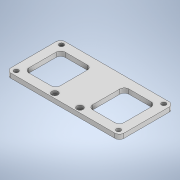
# Autodesk Inventor part: Battery_Plate
Saved by Autodesk Inventor 2021 (Build 250183000, 183)
## iProperties
Created: 2021-07-26
Part Number: Battery_Plate
Material: Generic
Document SubType Name: Modeling
Designer: rquic
Density: 1 g/cm^3
Appearance: Default
Author: rquic
Autodesk Inventor part; units mm, degrees
ref_plane "YZ Plane" through (0, 0, 0) normal (1, 0, 0) x (0, 1, 0)
ref_plane "XZ Plane" through (0, 0, 0) normal (0, 1, 0) x (-1, 0, 0)
ref_plane "XY Plane" through (0, 0, 0) normal (0, 0, 1) x (1, 0, 0)
sketch "Sketch1" plane through (0, 0, 0) normal (0, 1, 0) x (-1, 0, 0)
  line L0 (33.3375, 19.05) -> (-33.3375, 19.05)
  line L1 (-33.3375, 19.05) -> (-33.3375, -19.05)
  line L2 (-33.3375, -19.05) -> (33.3375, -19.05)
  line L3 (33.3375, -19.05) -> (33.3375, 19.05)
  line L4 (33.3375, 19.05) -> (-33.3375, -19.05) construction
  line L5 (-33.3375, 19.05) -> (33.3375, -19.05) construction
  line L6 (39.6875, -19.05) -> (-39.6875, -19.05)
  line L7 (-39.6875, -19.05) -> (-39.6875, 19.05)
  line L8 (-39.6875, 19.05) -> (39.6875, 19.05)
  line L9 (39.6875, 19.05) -> (39.6875, -19.05)
  line L10 (39.6875, -19.05) -> (-39.6875, 19.05) construction
  line L11 (-39.6875, -19.05) -> (39.6875, 19.05) construction
  circle A0 centre (35.8775, -15.875) radius 1.5875
  circle A1 centre (35.8775, 15.875) radius 1.5875
  circle A2 centre (-35.8775, -15.875) radius 1.5875
  circle A3 centre (-35.8775, 15.875) radius 1.5875
  line L12 (33.3375, 12.7) -> (-33.3375, 12.7)
  line L13 (-33.3375, 12.7) -> (-33.3375, -12.7)
  line L14 (-33.3375, -12.7) -> (33.3375, -12.7)
  line L15 (33.3375, -12.7) -> (33.3375, 12.7)
  line L16 (11.43, 12.7) -> (-11.43, 12.7)
  line L17 (-11.43, 12.7) -> (-11.43, -12.7)
  line L18 (-11.43, -12.7) -> (11.43, -12.7)
  line L19 (11.43, -12.7) -> (11.43, 12.7)
  circle A4 centre (8.8265, 15.875) radius 1.5875
  circle A5 centre (-8.8265, 15.875) radius 1.5875
  point P0 (0, 0)
  point P1 (0, 12.7)
  point P2 (0, 0)
  point P3 (0, 0)
  point P4 (0, -12.7)
  point P5 (0, 0)
  point P6 (-11.43, -12.7)
  point P7 (-11.43, 12.7)
  point P8 (11.43, -12.7)
  point P9 (11.43, 12.7)
  dimension "d0" = 66.675
  dimension "d1" = 38.1
  dimension "d2" = 6.35
  dimension "d5" = 31.75
  dimension "d8" = 71.755
  dimension "d11" = 2.54
  dimension "d12" = 3.175
  dimension "d14" = 3.175
  dimension "d15" = 66.675
  dimension "d19" = 22.86
  dimension "d23" = 3.175
  dimension "d24" = 3.175
  dimension "d25" = 17.653
  dimension "d26" = 8.8265
  dimension "d28" = 6.35
  dimension "d29" = 6.35
  constraints: 40 end point, 10 midpoint, 8 parallel, 6 centre point, 5 horizontal, 4 perpendicular, 2 collinear, 2 horizontal alignment, 2 vertical alignment, 1 vertical, 6 other
  measures "d0" distance of L1.end L2.end
  measures "d1" distance of L0.end L1.end
  measures "d2" distance between parallel lines of L1 L7
  measures "d5" distance of A0.centre A1.centre
  measures "d8" distance of A0.centre A2.centre
  measures "d11" distance from line of A0.centre L3
  measures "d12" distance from line of L2 A0.centre
  measures "d14" diameter of A1
  measures "d15" distance of L13.end L14.end
  measures "d19" distance of L16.start L16.end
  measures "d23" diameter of A4
  measures "d24" diameter of A5
  measures "d25" distance of A5.centre A4.centre
  measures "d26" horizontal distance of A4.centre point (0, 12.7)
  measures "d28" distance between parallel lines of L2 L14
  measures "d29" distance between parallel lines of L12 L8
extrude "Extrusion1" add sketch "Sketch1" along normal blind 3.175 contours L3 L12 L1 L0 | L8 L9 L6 L3 | L1 L6 L7 L8 | L3 L2 L1 L14 | L19 L14 L17 L12
fillet "Fillet1" radius 3.175 12 edges at (-39.6875, 1.5875, 19.05) (39.6875, 1.5875, 19.05) (-39.6875, 1.5875, -19.05) (39.6875, 1.5875, -19.05) (-33.3375, 1.5875, 12.7) (11.43, 1.5875, 12.7) (33.3375, 1.5875, 12.7) (11.43, 1.5875, -12.7) (33.3375, 1.5875, -12.7) (-11.43, 1.5875, -12.7) (-33.3375, 1.5875, -12.7) (-11.43, 1.5875, 12.7)
sketch "Sketch3" plane through (0, 3.175, 0) normal (0, 1, 0) x (1, 0, 0)
  circle A0 centre (-8.8265, -15.875) radius 1.5875 projected
  circle A1 centre (-8.8265, -15.875) radius 2.2225
  circle A2 centre (8.8265, -15.875) radius 1.5875 projected
  circle A3 centre (8.8265, -15.875) radius 2.2225
  point P0 (0, 0)
  dimension "d30" = 4.445
  dimension "d31" = 4.445
  constraints: 2 centre point, 2 coincident
  measures "d30" diameter of A1
  measures "d31" diameter of A3
extrude "Extrusion2" cut sketch "Sketch3" against normal blind 1.905 contours A0 | A1 | A2 | A3
equation "\"d15\" = d0"
equation "\"d23\" = d14"
equation "\"d24\" = d14"
equation "\"d26\" = 0.5 * d25"
equation "\"d28\" = d2"
equation "\"d29\" = d2"
body "Solid1"
